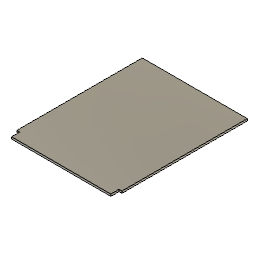
盖子 (Autodesk Fusion 360 design; units mm, degrees)
part number: 2025-10-22-10-29-16-926
Autodesk Fusion 360 part; units mm, degrees
sketch "Sketch1" plane through (0, 0, 0) normal (0, 0, 1) x (1, 0, 0)
  line L0 (50.828, 64.624) -> (-50.828, 64.624)
  line L1 (-50.828, 64.624) -> (-50.828, -64.624)
  line L2 (-50.828, -64.624) -> (50.828, -64.624)
  line L3 (50.828, -64.624) -> (50.828, 64.624)
  line L4 (50.828, 64.624) -> (-50.828, -64.624) construction
  line L5 (-50.828, 64.624) -> (50.828, -64.624) construction
  dimension "d1" = 101.656
  dimension "d2" = 129.248
  constraint horizontal L0
  constraint perpendicular L0 L1
  constraint parallel L0 L2
  constraint parallel L1 L3
  constraint coincident L4 origin
  constraint coincident L5 origin
  measures "d1" distance of L1.end L2.end
  measures "d2" distance of L0.end L1.end
extrude "Extrude1" add sketch "Sketch1" along normal blind 2
sketch "Sketch2" plane through (0, 0, 2) normal (0, 0, 1) x (-1, 0, 0)
  line L0 (-50.828, 64.624) -> (-50.828, -64.624)
  line L1 (-50.828, -64.624) -> (50.828, -64.624)
  line L2 (50.828, -64.624) -> (50.828, 64.624)
  line L3 (50.828, 64.624) -> (-50.828, 64.624)
  line L4 (0, 64.624) -> (0, -64.624) construction
  line L5 (-50.828, 64.624) -> (-48, 64.624) construction
  line L6 (-48, 64.624) -> (-48, 56.624)
  line L7 (-48, 56.624) -> (-50.828, 56.624)
  line L8 (-50.828, 56.624) -> (-50.828, 64.624) construction
  dimension "d5" = 2.828
  dimension "d6" = 8
  constraint midpoint L3 L4.start
  constraint midpoint L1 L4.end
  constraint horizontal L5
  constraint vertical L6
  constraint horizontal L7
  constraint vertical L8
  constraint coincident L0.start L3.end
  measures "d5" distance of L0.start L5.end
  measures "d6" distance of L0.start L7.end
extrude "Extrude2" cut sketch "Sketch2" against normal blind 2 contours L0 L3 L6 L7
mirror "Mirror1" about plane through (0, 0, 0) normal (1, 0, 0) of "Extrude2"
